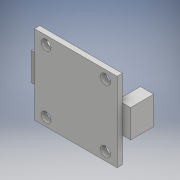
# Autodesk Inventor part: Mock Board
Saved by Autodesk Inventor 2017 (Build 210142000, 142)
## iProperties
Created: 2022-08-30
Part Number: Mock Board
Material: Generic
Document SubType Name: Modeling
Designer: Collin
Density: 1 g/cm^3
Appearance: Default
Author: Collin
## iProperties of the stored document Mock Board_3DPrint.ipt
Created: 2022-08-30
Part Number: Mock Board_3DPrint
Material: Generic
Document SubType Name: Modeling
Designer: Collin
Density: 1 g/cm^3
Appearance: Default
Author: Collin
Autodesk Inventor part; units mm, degrees
ref_plane "YZ Plane" through (0, 0, 0) normal (1, 0, 0) x (0, 1, 0)
ref_plane "XZ Plane" through (0, 0, 0) normal (0, 1, 0) x (-1, 0, 0)
ref_plane "XY Plane" through (0, 0, 0) normal (0, 0, 1) x (1, 0, 0)
sketch "Sketch1" plane through (0, 0, 0) normal (0, 1, 0) x (-1, 0, 0)
  line L0 (0, 0) -> (25, 0)
  line L1 (25, 0) -> (25, -24)
  line L2 (25, -24) -> (0, -24)
  line L3 (0, -24) -> (0, 0)
  dimension "d0" = 24
  dimension "d1" = 25
  constraints: 8 end point, 2 parallel, 1 horizontal, 1 perpendicular
  measures "d0" distance of L0.end L1.end
  measures "d1" distance of L0.start L0.end
extrude "Extrusion1" add sketch "Sketch1" along normal blind 1.6
sketch "Sketch2" plane through (0, 1.6, 0) normal (0, 1, 0) x (1, 0, 0)
  line L0 (-23.5, 7.75) -> (-27.5, 7.75)
  line L1 (-27.5, 7.75) -> (-27.5, 16.25)
  line L2 (-27.5, 16.25) -> (-23.5, 16.25)
  line L3 (-23.5, 16.25) -> (-23.5, 7.75)
  line L4 (-1.5, 7.75) -> (2.5, 7.75)
  line L5 (2.5, 7.75) -> (2.5, 16.25)
  line L6 (2.5, 16.25) -> (-1.5, 16.25)
  line L7 (-1.5, 16.25) -> (-1.5, 7.75)
  line L8 (-25, 0) -> (0, 0) projected
  line L9 (0, 24) -> (-25, 24) projected
  line L10 (0, 0) -> (0, 24) projected
  line L11 (-25, 24) -> (-25, 0) projected
  dimension "d4" = 8.5
  dimension "d5" = 7.75
  dimension "d6" = 7.75
  dimension "d8" = 4
  dimension "d9" = 8.5
  dimension "d10" = 7.75
  dimension "d11" = 2.5
  dimension "d13" = 4
  dimension "d14" = 2.5
  constraints: 16 end point, 4 parallel, 2 horizontal, 2 perpendicular
  measures "d4" distance of L0.end L1.end
  measures "d5" distance between parallel lines of L8 L0
  measures "d6" distance between parallel lines of L9 L2
  measures "d8" distance of L5.end L6.end
  measures "d9" distance of L6.end L4.start
  measures "d10" distance between parallel lines of L8 L4
  measures "d11" distance between parallel lines of L10 L5
  measures "d13" distance between parallel lines of L3 L1
  measures "d14" distance between parallel lines of L11 L1
extrude "Extrusion2" add sketch "Sketch2" along normal blind 7 contours L0 L11 L2 L3 | L0 L1 L2 L11 | L10 L6 L5 L4 | L4 L7 L6 L10
sketch "Sketch3" plane through (0, 1.6, 0) normal (0, 1, 0) x (1, 0, 0)
  line L0 (-25, 7.75) -> (-25, 0) projected
  line L1 (-25, 0) -> (0, 0) projected
  point P0 (-21.5, 2.5)
  point P1 (-21.5, 21.5)
  point P2 (-3.5, 2.5)
  point P3 (-3.5, 21.5)
  dimension "d17" = 3.5
  dimension "d18" = 2.5
  dimension "d21" = 19
  dimension "d24" = 18
  constraints: 1 horizontal, 1 vertical, 3 other
  measures "d17" distance from line of L0 point (-21.5, 2.5)
  measures "d18" distance from line of L1 point (-21.5, 2.5)
  measures "d21" distance of point (-21.5, 2.5) point (-21.5, 21.5)
  measures "d24" distance of point (-21.5, 2.5) point (-3.5, 2.5)
hole "Hole1" at (-21.5, 1.6, -2.5) at (-21.5, 1.6, -21.5) at (-3.5, 1.6, -2.5) at (-3.5, 1.6, -21.5) direction (0, -1, 0) diameter 3 end through all
body "Solid1"
